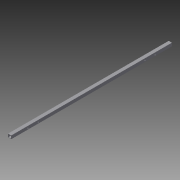
# Autodesk Inventor part: 1inSquareSupport2
Saved by Autodesk Inventor 2015 SP1 (Build 190203100, 203)
## iProperties
Created: 2016-03-21
Part Number: 1inSquareSupport2
Material: Generic
Document SubType Name: Modeling
Designer: Mac
Density: 1 g/cm^3
Appearance: Default
L: 50.000 in
thick: 0.120 in
Author: Mac
Autodesk Inventor part; units mm, degrees
ref_plane "YZ Plane" through (0, 0, 0) normal (1, 0, 0) x (0, 1, 0)
ref_plane "XZ Plane" through (0, 0, 0) normal (0, 1, 0) x (-1, 0, 0)
ref_plane "XY Plane" through (0, 0, 0) normal (0, 0, 1) x (1, 0, 0)
sketch "Sketch1" plane through (0, 0, 0) normal (0, 0, 1) x (1, 0, 0)
  line L0 (-12.7, 12.7) -> (12.7, 12.7)
  line L1 (12.7, 12.7) -> (12.7, -12.7)
  line L2 (12.7, -12.7) -> (-12.7, -12.7)
  line L3 (-12.7, -12.7) -> (-12.7, 12.7)
  line L4 (9.652, 9.652) -> (-9.652, 9.652)
  line L5 (-9.652, 9.652) -> (-9.652, -9.652)
  line L6 (-9.652, -9.652) -> (9.652, -9.652)
  line L7 (9.652, -9.652) -> (9.652, 9.652)
  point P0 (0, 0)
  point P1 (0, 12.7)
  point P2 (12.7, 0)
  point P3 (-12.7, 0)
  dimension "d0" = 25.4
  dimension "d1" = 25.4
  dimension "d2" = 3.048
  constraints: 16 end point, 4 parallel, 3 midpoint, 2 perpendicular, 1 horizontal, 1 horizontal alignment, 1 vertical alignment, 3 other
  measures "d0" distance of L0.start L0.end
  measures "d1" distance of L0.end L1.end
  measures "d2" distance between parallel lines of L4 L0
extrude "Extrusion1" add sketch "Sketch1" along normal mid plane 1270
sketch "Sketch2" plane through (12.7, 12.7, 635) normal (1, 0, 0) x (0, 0, -1)
  circle A0 centre (132.7, -12.693) radius 4.25 projected
  circle A1 centre (212.7, -12.693) radius 4.25 projected
  circle A2 centre (1057.3, -12.693) radius 4.25 projected
  circle A3 centre (1137.3, -12.693) radius 4.25 projected
  point P0 (635, -12.7)
  constraints: 4 coincident
hole "Hole1" at (12.7, 0.007, 502.3) at (12.7, 0.007, 422.3) at (12.7, 0.007, -422.3) at (12.7, 0.007, -502.3) direction (-1, 0, 0) diameter 6.7564 depth 12.7 tip angle 118
sketch "Sketch3" plane through (-12.7, -12.7, -635) normal (-1, 0, 0) x (0, 0, 1)
  point P0 (635, 12.7)
equation "\"d2\" = thick"
equation "\"d3\" = L"
equation "\"L\" = 1270"
equation "\"thick\" = 3.048"
body "Solid1"
